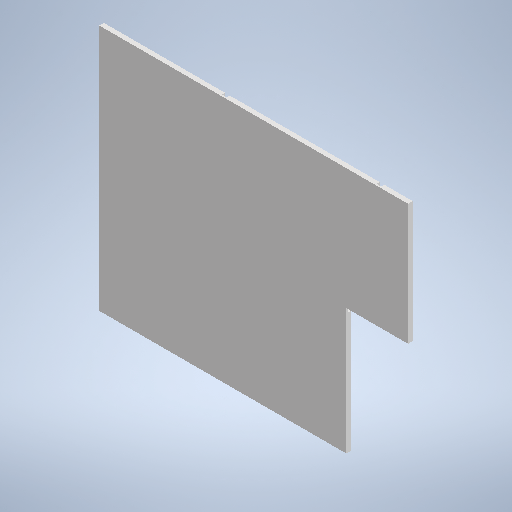
# Autodesk Inventor part: Wire Position
Saved by Autodesk Inventor 2025.2 (Build 292293000, 293)
## iProperties
Created: 2025-04-29
Part Number: Wire Position
Material: Generic
Document SubType Name: Modeling
Designer: powel
Density: 1 g/cm^3
Appearance: Default
Author: powel
Autodesk Inventor part; units mm, degrees
ref_plane "YZ Plane" through (0, 0, 0) normal (1, 0, 0) x (0, 1, 0)
ref_plane "XZ Plane" through (0, 0, 0) normal (0, 1, 0) x (-1, 0, 0)
ref_plane "XY Plane" through (0, 0, 0) normal (0, 0, 1) x (1, 0, 0)
sketch "Sketch1" plane through (0, 0, 0) normal (0, 0, 1) x (1, 0, 0)
  line L0 (0, 0) -> (32, 0)
  line L1 (32, 0) -> (32, 32)
  line L2 (32, 32) -> (0, 32)
  line L3 (0, 32) -> (0, 0)
  line L4 (0, 16) -> (0, 15.7)
  line L5 (0, 15.7) -> (0, 16.3)
  line L6 (32, 16.3) -> (32, 15.7)
  line L7 (0, 15.7) -> (0, 16.3)
  line L8 (16.3, 16.3) -> (16.3, 32)
  line L9 (16.3, 32) -> (15.7, 32)
  line L10 (15.7, 32) -> (15.7, 16.3)
  line L11 (15.7, 32) -> (16.3, 32)
  line L12 (16.3, 0) -> (15.7, 0)
  line L13 (0, 16.3) -> (15.7, 16.3)
  line L14 (16.3, 16.3) -> (32, 16.3)
  line L15 (32, 15.7) -> (16.3, 15.7)
  line L16 (15.7, 15.7) -> (0, 15.7)
  line L17 (16.3, 32) -> (16.3, 16.3)
  line L18 (16.3, 15.7) -> (16.3, 0)
  line L19 (15.7, 0) -> (15.7, 15.7)
  line L20 (15.7, 16.3) -> (15.7, 32)
  line L21 (32, 16.3) -> (40, 16.3)
  line L22 (40, 16.3) -> (40, 32)
  line L23 (40, 32) -> (32, 32)
  line L24 (32, 32) -> (32, 16.3)
  line L25 (36, 32) -> (35.7, 32)
  line L26 (35.7, 32) -> (36.3, 32)
  line L27 (36.3, 32) -> (36.3, 16.3)
  line L28 (36.3, 16.3) -> (35.7, 16.3)
  line L29 (35.7, 16.3) -> (35.7, 32)
  dimension "d0" = 32
  dimension "d1" = 32
  dimension "d2" = 0.3
  dimension "d3" = 0.6
  dimension "d4" = 0.6
  dimension "d6" = 0.6
  dimension "d7" = 8
  dimension "d8" = 0.3
  dimension "d9" = 0.6
  constraints: 60 end point, 17 parallel, 7 perpendicular, 7 point on line, 6 horizontal, 2 midpoint
  measures "d0" distance of L2.end L1.end
  measures "d1" distance of L2.end L0.start
  measures "d2" distance of L4.start L4.end
  measures "d3" distance of L4.end L5.end
  measures "d4" distance of L6.start L6.end
  measures "d6" distance of L9.end L8.end
  measures "d7" distance of L23.end L22.end
  measures "d8" distance of L25.start L25.end
  measures "d9" distance of L27.end L28.end
extrude "Extrusion1" add sketch "Sketch1" against normal blind 0.4 contours L3 L16 L19 L0 | L18 L15 L1 L0 | L3 L2 L10 L13 | L14 L8 L2 L1 | L1 L23 L29 L21 | L27 L23 L22 L21
extrude "Extrusion2" add sketch "Sketch1" along normal blind 0.2
body "Solid1"
